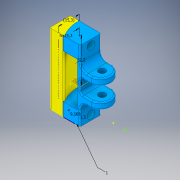
# Autodesk Inventor part: pedal_adapter
Saved by Autodesk Inventor 2019 (Build 230136000, 136)
## iProperties
Created: 2021-05-24
Part Number: pedal_adapter
Material: Genérico
Document SubType Name: Modeling
Designer: Juan M. Casillas
Density: 1 g/cm^3
Appearance: Valor por defecto
Author: Juan M. Casillas
## iProperties of the stored document pedal_adapter_3DPrint.ipt
Created: 2021-05-24
Part Number: pedal_adapter_3DPrint
Material: Genérico
Document SubType Name: Modeling
Designer: Juan M. Casillas
Density: 1 g/cm^3
Appearance: Valor por defecto
Author: Juan M. Casillas
Autodesk Inventor part; units mm, degrees
ref_plane "YZ Plane" through (0, 0, 0) normal (1, 0, 0) x (0, 1, 0)
ref_plane "XZ Plane" through (0, 0, 0) normal (0, 1, 0) x (-1, 0, 0)
sketch "Sketch1" plane through (0, 0, 0) normal (0, 1, 0) x (-1, 0, 0)
  line L0 (3.25, 7.8514) -> (-1.8413, 7.8514) construction
  line L1 (-1.8413, 7.8514) -> (6.3293, 7.8514)
  line L2 (7.3293, 6.8514) -> (7.3293, -6.4486)
  line L3 (6.3293, -7.4486) -> (1.9313, -7.4486)
  line L4 (-3.6707, 7.8514) -> (0.9293, -7.4486) construction
  line L5 (7.3293, 7.8514) -> (7.3293, -7.4486) construction
  line L6 (7.3293, 7.8514) -> (7.3293, 0.2014) construction
  line L7 (7.3293, 0.2014) -> (-1.2707, 0.2014) construction
  arc A0 (0.9314, -6.4654) -> (-2.701, 6.3407) centre (-24.9911, -6.9001) ccw
  arc A1 (7.3293, 6.8514) -> (6.3293, 7.8514) centre (6.3293, 6.8514) ccw
  arc A2 (6.3293, -7.4486) -> (7.3293, -6.4486) centre (6.3293, -6.4486) ccw
  arc A3 (0.9314, -6.4654) -> (1.9313, -7.4486) centre (1.9313, -6.4486) ccw
  arc A4 (-1.8413, 7.8514) -> (-2.701, 6.3407) centre (-1.8413, 6.8514) ccw
  point P0 (0, 0)
  point P1 (-1.3707, 0.2014)
  dimension "d2" = 11
  dimension "d3" = 15.3
  dimension "d4" = 6.4
  dimension "d5" = 7.65
  dimension "d7" = 1
  constraints: 16 end point, 13 point on circle, 8 tangent, 7 point on line, 5 centre point, 3 equal radius, 2 horizontal, 2 midpoint, 1 collinear, 1 perpendicular, 1 vertical
  measures "d2" distance of L4.start L5.start
  measures "d3" distance of L5.start L5.end
  measures "d4" distance of L5.end L4.end
  measures "d5" distance of L5.start L6.end
  measures "d7" radius of A1
extrude "Extrusion1" add sketch "Sketch1" along normal blind 52
ref_plane "Work Plane1" through (-0.9293, 0, -6.4486) normal (-1, 0, 0) x (0, 0, 1)
sketch "Sketch2" plane through (-0.9293, 0, -6.4486) normal (-1, 0, 0) x (0, 0, 1)
  line L0 (13.3, 0) -> (0, 0) construction
  line L1 (13.3, 0) -> (13.3, 52) construction
  line L2 (0, 52) -> (13.3, 52) construction
  line L3 (0, 0) -> (0, 52) construction
  line L4 (6.4486, 0) -> (6.4486, 52) construction
  line L5 (0, 52) -> (13.3, 52) construction
  line L6 (13.3, 0) -> (13.3, 52) construction
  line L7 (13.3, 26) -> (0, 26) construction
  line L8 (6.4486, 0) -> (6.4486, 10) construction
  line L9 (6.4486, 52) -> (6.4486, 42) construction
  point P0 (6.4486, 4)
  point P1 (6.4486, 48)
  point P2 (6.4486, 4)
  point P3 (6.4486, 48)
  dimension "d12" = 10
  dimension "d13" = 10
  constraints: 8 end point, 5 point on line, 2 coincident, 2 midpoint, 1 perpendicular, 4 other
  measures "d12" distance of L4.start L8.end
  measures "d13" distance of L4.end L9.end
hole "Hole1" at (-0.9293, 4, 0) at (-0.9293, 48, 0) direction (-1, 0, 0) diameter 2.95 end through all both
sketch "Sketch3" plane through (0, 0, 0) normal (0, -1, 0) x (1, 0, 0)
  arc A0 (2.701, 6.3407) -> (-0.9314, -6.4654) centre (24.9911, -6.9001) ccw projected
  arc A1 (-1.9313, -7.4486) -> (-0.9314, -6.4654) centre (-1.9313, -6.4486) ccw projected
  line L0 (1.8413, 7.8514) -> (-6.3293, 7.8514) construction
  line L1 (-6.3293, -7.4486) -> (-1.9313, -7.4486) construction
  arc A2 (-0.9314, -6.4654) -> (-0.8972, -7.4486) centre (12.1076, -6.5033) ccw construction
  arc A3 (12.2289, 6.3407) -> (8.5968, -6.4648) centre (34.5193, -6.8995) ccw
  arc A4 (7.0968, -6.4648) -> (7.0967, -6.4653) centre (33.0193, -6.8995) ccw
  arc A5 (-1.9313, -7.4486) -> (-0.9314, -6.4654) centre (-1.9313, -6.4486) ccw projected
  line L2 (7.5947, -7.4486) -> (-1.0269, -7.4486)
  arc A6 (2.701, 6.3407) -> (1.8413, 7.8514) centre (1.8413, 6.8514) ccw projected
  line L3 (11.3708, 7.8514) -> (2.6198, 7.8514)
  arc A7 (12.2289, 6.3407) -> (11.3708, 7.8514) centre (11.3691, 6.8514) ccw
  arc A8 (7.5947, -7.4486) -> (8.5968, -6.4648) centre (7.5969, -6.4486) ccw
  arc A9 (2.6198, 7.8514) -> (2.5021, 7.602) centre (2.6198, 7.6989) ccw
  arc A10 (-1.1844, -7.1136) -> (-1.0269, -7.4486) centre (-1.0269, -7.244) ccw
  line L4 (9.577, 0.175) -> (11.077, 0.175) construction
  point P0 (0, 0)
  point P1 (7.0989, -7.4486)
  point P2 (1, 1)
  point P3 (0.069, -5.439)
  point P4 (0.069, 0.2453)
  dimension "d25" = 1
  dimension "d36" = 9.508
  dimension "d37" = 1.5
  constraints: 16 point on circle, 6 centre point, 6 end point, 4 tangent, 3 horizontal, 2 point on line, 1 equal radius, 6 other
  measures "d25" radius of A7
  measures "d36" horizontal distance of point (0.069, 0.245) L4.start
  measures "d37" distance of L4.start L4.end
sketch "Sketch5" plane through (-0.9293, 0, -6.4486) normal (-1, 0, 0) x (0, 0, 1)
  line L0 (-1, 0) -> (-1, 52) construction
  line L1 (0, 52) -> (13.3, 52) construction
  line L2 (14.3, 0) -> (14.3, 52) construction
  line L3 (13.3, 0) -> (0, 0) construction
  line L4 (13.3, 0) -> (14.3, 0) construction
  line L5 (0, 0) -> (-1, 0) construction
  line L6 (0, 52) -> (-1, 52) construction
  line L7 (14.3, 52) -> (13.3, 52) construction
  line L8 (6.65, 52) -> (6.65, 0) construction
  line L9 (6.65, 26) -> (14.3, 26) construction
  line L10 (6.65, 26) -> (-1, 26) construction
  line L11 (14.3, 9.9) -> (-1, 9.9) construction
  line L12 (-1, 9.9) -> (-1, 42.1) construction
  line L13 (-1, 42.1) -> (14.3, 42.1) construction
  line L14 (14.3, 42.1) -> (14.3, 9.9) construction
  line L15 (14.3, 9.9) -> (-1, 42.1) construction
  line L16 (-1, 9.9) -> (14.3, 42.1) construction
  point P0 (6.4486, 0)
  point P1 (6.65, 9.9)
  point P2 (6.65, 42.1)
  dimension "d30" = 32.2
  dimension "d31" = 15.3
  dimension "d32" = 15.3
  constraints: 26 end point, 9 midpoint, 5 equal length, 2 perpendicular, 1 coincident, 1 horizontal
  measures "d30" distance of L11.end L12.end
  measures "d31" distance of L12.end L13.end
  measures "d32" distance of L0.end L2.end
extrude "Extrusion3" add sketch "Sketch3" against normal up to surface (9.9 mm away) separate body contours A6 A9 L3 A7 A4 L2 A10 A1 A0 | A4 A7 A3 A8 L2 picked at (8.5645, -0.3371)
sketch "Sketch6" plane through (2.6198, 9.9, 7.8514) normal (0, 1, 0) x (1, 0, 0)
  arc A0 (5.977, 14.3162) -> (9.6091, 1.5107) centre (31.8995, 14.751) ccw projected
  line L0 (4.9749, 15.3) -> (-3.6467, 15.3) construction
  line L1 (0, 0) -> (8.751, 0) construction
  line L2 (4.9749, 15.3) -> (9.369, 15.3)
  line L3 (8.751, 0) -> (0, 0) construction
  line L4 (8.751, 0) -> (12.7005, 0)
  arc A1 (5.977, 14.3162) -> (9.6091, 1.5107) centre (31.8995, 14.751) ccw construction
  line L5 (5.9791, 15.3) -> (6.9791, 15.3) construction
  line L6 (10.5787, 0) -> (12.5787, 0) construction
  line L7 (12.5787, 0) -> (12.5787, 15.3)
  line L8 (12.5787, 15.3) -> (5.9791, 15.3)
  arc A2 (5.977, 14.3162) -> (4.9749, 15.3) centre (4.9771, 14.3) ccw projected
  arc A3 (8.751, 0) -> (9.6091, 1.5107) centre (8.7493, 1) ccw projected
  point P0 (-2.6198, 7.8514)
  dimension "d38" = 1
  dimension "d39" = 2
  constraints: 12 end point, 5 point on line, 2 point on circle, 1 horizontal, 1 perpendicular, 1 vertical
  measures "d38" distance of L5.start L5.end
  measures "d39" distance of L6.start L6.end
extrude "Extrusion4" add sketch "Sketch6" against normal up to surface (9.9 mm away) bodies 2
extrude "Extrusion6" add sketch "Sketch6" along normal up to surface (16.1 mm away) bodies 2
sketch "Sketch7" plane through (7.5947, 26, -7.4486) normal (0, 1, 0) x (1, 0, 0)
  arc A0 (1.0021, -0.9838) -> (4.6342, -13.7893) centre (26.9246, -0.549) ccw projected
  line L0 (0, 0) -> (7.6039, 0) projected
  line L1 (7.6039, -15.3) -> (3.7762, -15.3) projected
  line L2 (-8.6216, 0) -> (7.6039, 0) projected
  arc A1 (1.0021, -0.9838) -> (0, 0) centre (0.0022, -1) ccw projected
  arc A2 (1.0043, 0) -> (1.0021, -0.9838) centre (26.9246, -0.5488) ccw
  line L3 (7.6039, -15.3) -> (-4.9749, -15.3) projected
  arc A3 (4.6342, -13.7893) -> (5.604, -15.3) centre (26.9799, -0.5115) ccw
  arc A4 (3.7762, -15.3) -> (4.6342, -13.7893) centre (3.7745, -14.3) ccw projected
  point P0 (-7.5947, -7.4486)
  constraints: 5 point on circle, 2 centre point, 2 point on line
extrude "Extrusion7" cut sketch "Sketch7" against normal up to surface (16.1 mm away) bodies 2
sketch "Sketch8" plane through (15.1985, 0, 7.8514) normal (1, 0, 0) x (0, 0, -1)
  point P0 (7.8514, 0)
  point P1 (7.8514, 4)
  constraints: 1 other
hole "Hole2" at (15.1985, 4, 0) direction (-1, 0, 0) diameter 2.85 end through all counterbore diameter 5.65 counterbore depth 10 bodies 2
ref_plane "Work Plane4" through (15.1985, 26, 7.8514) normal (0, 1, 0) x (1, 0, 0)
mirror "Mirror1" about plane through (15.1985, 26, 7.8514) normal (0, 1, 0) bodies 2
sketch "Sketch10" plane through (15.1985, 0, 7.8514) normal (1, 0, 0) x (0, 0, -1)
  circle A0 centre (7.8514, 48) radius 2.825 construction
  circle A1 centre (7.8514, 4) radius 2.825 construction
  line L0 (0, 0) -> (15.3, 0) construction
  line L1 (15.3, 52) -> (15.3, 0) construction
  line L2 (0, 52) -> (15.3, 52) construction
  line L3 (0, 52) -> (0, 0) construction
  line L4 (14.3, 52) -> (1, 52) construction
  line L5 (7.65, 52) -> (7.65, 0) construction
  line L6 (1, 0) -> (14.3, 0) construction
  line L7 (0, 0) -> (0, 52) construction
  line L8 (15.3, 21) -> (0, 21) construction
  line L9 (0, 21) -> (0, 31) construction
  line L10 (0, 31) -> (15.3, 31) construction
  line L11 (15.3, 31) -> (15.3, 21) construction
  line L12 (15.3, 21) -> (0, 31) construction
  line L13 (0, 21) -> (15.3, 31) construction
  line L14 (15.3, 20.85) -> (0, 20.85)
  line L15 (0, 20.85) -> (0, 31.15)
  line L16 (0, 31.15) -> (15.3, 31.15)
  line L17 (15.3, 31.15) -> (15.3, 20.85)
  line L18 (15.3, 20.85) -> (0, 31.15) construction
  line L19 (0, 20.85) -> (15.3, 31.15) construction
  line L20 (15.3, 20.85) -> (0, 20.85)
  line L21 (0, 20.85) -> (0, 15.85)
  line L22 (0, 15.85) -> (15.3, 15.85)
  line L23 (15.3, 15.85) -> (15.3, 20.85)
  line L24 (15.3, 31.15) -> (0, 31.15)
  line L25 (0, 31.15) -> (0, 36.15)
  line L26 (0, 36.15) -> (15.3, 36.15)
  line L27 (15.3, 36.15) -> (15.3, 31.15)
  point P0 (7.8514, 0)
  point P1 (7.65, 26)
  dimension "d56" = 10
  dimension "d57" = 10.3
  dimension "d58" = 5
  dimension "d59" = 5
  constraints: 42 end point, 8 parallel, 7 midpoint, 4 horizontal, 4 perpendicular, 4 point on line
  measures "d56" distance of L8.end L9.end
  measures "d57" distance of L14.end L15.end
  measures "d58" distance of L21.end L20.end
  measures "d59" distance of L24.end L25.end
extrude "Extrusion8" add sketch "Sketch10" along normal blind 15 contours L23 L22 L21 L14 | L16 L25 L26 L27 bodies 2
sketch "Sketch11" plane through (15.1985, 15.85, -7.4486) normal (0, -1, 0) x (1, 0, 0)
  line L0 (15, 15.3) -> (15, 0) construction
  line L1 (15, 7.65) -> (11, 7.65) construction
  line L2 (11, 7.65) -> (8.5, 7.65) construction
  circle A0 centre (8.5, 7.65) radius 2.5
  point P0 (-15.1985, 7.4486)
  dimension "d62" = 4
  dimension "d63" = 2.5
  constraints: 4 end point, 2 horizontal, 1 coincident, 1 horizontal alignment, 1 midpoint, 2 other
  measures "d62" distance of L1.start L1.end
  measures "d63" distance of L1.end L2.end
extrude "Extrusion9" cut sketch "Sketch11" against normal through all bodies 2
sketch "Sketch12" plane through (15.1985, 15.85, -7.4486) normal (0, -1, 0) x (1, 0, 0)
  point P0 (-15.1985, 7.4486)
sketch "Sketch13" plane through (15.1985, 15.85, -7.4486) normal (0, -1, 0) x (1, 0, 0)
  circle A0 centre (8.5, 7.65) radius 2.5 construction
  line L0 (0, 0) -> (0, 15.3) construction
  line L1 (15, 15.3) -> (15, 0) projected
  line L2 (8.5, 15.3) -> (8.5, 0) construction
  line L3 (0, 0) -> (15, 0) construction
  arc A1 (8.5, 0) -> (8.5, 15.3) centre (7.2483, 7.65) ccw
  line L4 (0, 15.3) -> (15, 15.3)
  line L5 (8.5, 15.3) -> (15, 15.3) construction
  line L6 (15, 0) -> (15, 15.3) construction
  line L7 (15, 15.3) -> (15, 0) construction
  line L8 (15, 0) -> (8.5, 0) construction
  line L9 (8.5, 15.3) -> (15, 15.3)
  line L10 (15, 15.3) -> (15, 0)
  line L11 (15, 0) -> (8.5, 0)
  point P0 (-15.1985, 7.4486)
  point P1 (15, 7.65)
  constraints: 16 end point, 3 collinear, 3 point on circle, 2 centre point, 2 perpendicular, 1 midpoint, 1 point on line
extrude "Extrusion10" cut sketch "Sketch13" against normal through all bodies 2
fillet "Fillet1" radius 5 2 edges at (15.1985, 36.15, 0.2014) (15.1985, 15.85, 0.2014)
fillet "Fillet2" radius 2 2 edges at (15.1985, 31.15, 0.2014) (15.1985, 20.85, 0.2014)
fillet "Fillet3" radius 1 14 edges at (21.9485, 36.15, 7.8514) (30.1985, 36.15, 0.2014) (21.9485, 36.15, -7.4486) (16.663, 37.6145, 7.8514) (15.1985, 46.575, 7.8514) (16.663, 37.6145, -7.4486) (15.1985, 46.575, -7.4486) (21.9485, 15.85, -7.4486) (30.1985, 15.85, 0.2014) (21.9485, 15.85, 7.8514) (16.663, 14.3855, -7.4486) (15.1985, 5.425, -7.4486) (16.663, 14.3855, 7.8514) (15.1985, 5.425, 7.8514)
fillet "Fillet4" radius 1 12 edges at (30.1985, 31.15, 0.2014) (15.7843, 30.5642, 7.8514) (15.1985, 26, 7.8514) (15.7843, 21.4358, 7.8514) (20.4485, 20.85, 7.8514) (20.4485, 31.15, 7.8514) (30.1985, 20.85, 0.2014) (15.7843, 21.4358, -7.4486) (20.4485, 20.85, -7.4486) (15.7843, 30.5642, -7.4486) (20.4485, 31.15, -7.4486) (15.1985, 26, -7.4486)
equation "\"d31\" = d32"
body "Solid1"
body "Solid3"
